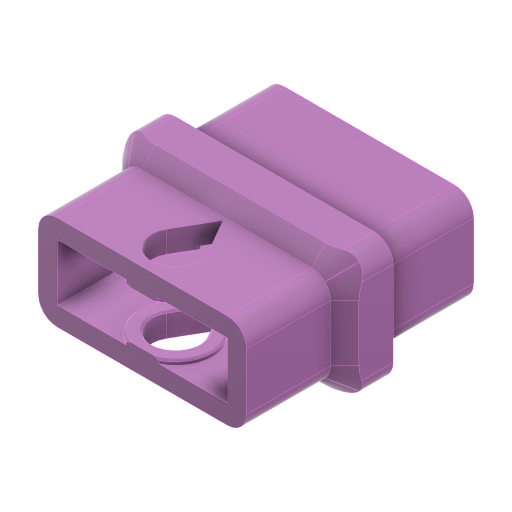
# Autodesk Inventor part: Короб подшипника
Saved by Autodesk Inventor 2024.1 (Build 281209000, 209)
## iProperties
Created: 2023-06-09
Part Number: Короб подшипника
Material: Типовые
Document SubType Name: Modeling
Designer: Admin
Density: 1 g/cm^3
Appearance: По умолчанию
Author: Admin
Autodesk Inventor part; units mm, degrees
ref_plane "YZ Plane" through (0, 0, 0) normal (1, 0, 0) x (0, 1, 0)
ref_plane "XZ Plane" through (0, 0, 0) normal (0, 1, 0) x (-1, 0, 0)
ref_plane "XY Plane" through (0, 0, 0) normal (0, 0, 1) x (1, 0, 0)
sketch "Эскиз1" plane through (0, 0, 0) normal (0, 0, 1) x (1, 0, 0)
  line L0 (-9, -5) -> (9, -5)
  line L1 (11, -3) -> (11, 3)
  line L2 (9, 5) -> (-9, 5)
  line L3 (-11, 3) -> (-11, -3)
  line L4 (-11, -5) -> (11, 5) construction
  line L5 (11, -5) -> (-11, 5) construction
  line L6 (-9, -3) -> (9, -3)
  line L7 (9, -3) -> (9, 3)
  line L8 (9, 3) -> (-9, 3)
  line L9 (-9, 3) -> (-9, -3)
  line L10 (-9, -3) -> (9, 3) construction
  line L11 (9, -3) -> (-9, 3) construction
  line L12 (-10.5, 6.5) -> (10.5, 6.5)
  line L13 (12.5, 4.5) -> (12.5, -4.5)
  line L14 (10.5, -6.5) -> (-10.5, -6.5)
  line L15 (-12.5, -4.5) -> (-12.5, 4.5)
  arc A0 (-9, 5) -> (-11, 3) centre (-9, 3) ccw
  arc A1 (-11, -3) -> (-9, -5) centre (-9, -3) ccw
  arc A2 (9, -5) -> (11, -3) centre (9, -3) ccw
  arc A3 (11, 3) -> (9, 5) centre (9, 3) ccw
  arc A4 (-10.5, 6.5) -> (-12.5, 4.5) centre (-10.5, 4.5) ccw
  arc A5 (-12.5, -4.5) -> (-10.5, -6.5) centre (-10.5, -4.5) ccw
  arc A6 (10.5, -6.5) -> (12.5, -4.5) centre (10.5, -4.5) ccw
  arc A7 (12.5, 4.5) -> (10.5, 6.5) centre (10.5, 4.5) ccw
  point P0 (0, 0)
  dimension "d0" = 1.5
  dimension "d1" = 18
  dimension "d2" = 6
  dimension "d5" = 2
  constraints: 32 end point, 16 point on circle, 16 tangent, 8 centre point, 8 point on line, 7 equal radius, 6 parallel, 4 midpoint, 3 perpendicular, 2 horizontal, 1 horizontal alignment, 1 vertical alignment, 3 other
  measures "d0" distance between parallel lines of L2 L12
  measures "d1" distance of L7.end L8.end
  measures "d2" distance of L6.end L7.end
  measures "d5" radius of A0
extrude "Выдавливание1" add sketch "Эскиз1" along normal blind 14 and the other way blind 10 contours A1 L3 A0 L2 A3 L1 A2 L0
extrude "Выдавливание2" add sketch "Эскиз1" along normal blind 3 contours L12 A7 L13 A6 L14 A5 L15 A4
sketch "Эскиз2" plane through (0, 0, -10) normal (0, 0, -1) x (-1, 0, 0)
  line L0 (9, -3) -> (-9, -3) projected
  line L1 (9, 3) -> (9, -3) projected
  line L2 (-9, 3) -> (9, 3) projected
  line L3 (-9, -3) -> (-9, 3) projected
  point P0 (0, 0)
extrude "Выдавливание3" add sketch "Эскиз2" against normal blind 3
fillet "Сопряжение1" radius 9 2 edges at (9, 0, -7) (-9, 0, -7)
sketch "Эскиз3" plane through (-9, 5, 14) normal (0, 1, 0) x (1, 0, 0)
  circle A0 centre (9, 3.5) radius 2.5
  line L0 (11.1651, 4.75) -> (9, 8.5)
  line L1 (9, 8.5) -> (6.8349, 4.75)
  line L2 (18, 0) -> (0, 0) projected
  line L3 (13, 5.8094) -> (13, 1.1906) construction
  line L4 (13, 1.1906) -> (9, -1.1188) construction
  line L5 (9, -1.1188) -> (5, 1.1906) construction
  line L6 (5, 1.1906) -> (5, 5.8094) construction
  line L7 (5, 5.8094) -> (9, 8.1188) construction
  line L8 (9, 8.1188) -> (13, 5.8094) construction
  point P0 (9, 14)
  point P1 (9, 0)
  dimension "d16" = 60
  dimension "d17" = 3.5
  dimension "d18" = 8
  constraints: 16 end point, 2 point on circle, 2 tangent, 2 vertical alignment, 1 centre point, 1 coincident, 1 midpoint, 1 vertical, 14 other
  measures "d16" angle of L0 L1
  measures "d17" distance from line of L2 A0.centre
  measures "d18" distance between parallel lines of L6 L3
chamfer "Фаска1" distance 2.121 angle 45 8 edges at (10.4142, 4.4142, 3) (0, 5, 3) (-10.4142, 4.4142, 3) (-11, 0, 3) (-10.4142, -4.4142, 3) (0, -5, 3) (10.4142, -4.4142, 3) (11, 0, 3)
extrude "Выдавливание4" cut sketch "Эскиз3" against normal through all
sketch "Эскиз4" plane through (-9, 3, 14) normal (0, -1, 0) x (1, 0, 0)
  circle A0 centre (9, -3.5) radius 3.9
  arc A1 (11.1651, -4.75) -> (6.8349, -4.75) centre (9, -3.5) ccw projected
  line L0 (0, 0) -> (18, 0) projected
  line L1 (9, -8.5) -> (6.8349, -4.75) projected
  line L2 (11.1651, -4.75) -> (9, -8.5) projected
  point P0 (9, -14)
  point P1 (9.6684, -7.3423)
  point P2 (10.7205, 0)
  point P3 (7.2795, 0)
  point P4 (8.3316, -7.3423)
  constraints: 1 centre point, 1 coincident, 1 other
extrude "Выдавливание5" add sketch "Эскиз4" along normal blind 0.5 contours A0 L2 A1 L1 L0
fillet "Сопряжение2" radius 0.25 2 edges at (-0.6684, 2.75, 6.6577) (0.6684, 2.75, 6.6577)
chamfer "Фаска2" distance 0.2 angle 45 7 edges at (-3.8921, 2.5, 10.2521) (-0.9885, 2.5, 6.8877) (-1.5651, 2.5, 8.2108) (0, 2.5, 13) (1.5651, 2.5, 8.2108) (0.9885, 2.5, 6.8877) (3.8921, 2.5, 10.2521)
mirror "Зеркальное отражение2" about plane through (0, 0, 0) normal (0, 1, 0) of "Выдавливание5", "Фаска2", "Сопряжение2"
